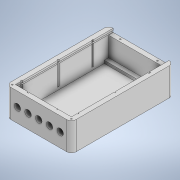
# Autodesk Inventor part: carcasa inferior
Saved by Autodesk Inventor 2020 (Build 240168000, 168)
## iProperties
Created: 2022-05-20
Part Number: carcasa inferior
Material: Generic
Document SubType Name: Modeling
Designer: juanc
Density: 1 g/cm^3
Appearance: Default
Author: juanc
## iProperties of the stored document _3DPrint.ipt
Created: 2022-05-23
Part Number: _3DPrint
Material: Generic
Document SubType Name: Modeling
Designer: juanc
Density: 1 g/cm^3
Appearance: Default
Author: juanc
Autodesk Inventor part; units mm, degrees
ref_plane "YZ Plane" through (0, 0, 0) normal (1, 0, 0) x (0, 1, 0)
ref_plane "XZ Plane" through (0, 0, 0) normal (0, 1, 0) x (-1, 0, 0)
sketch "Sketch1" plane through (0, 0, 0) normal (0, 1, 0) x (-1, 0, 0)
  line L0 (0, 0) -> (60, 0)
  line L1 (60, 0) -> (60, -100)
  line L2 (60, -100) -> (0, -100)
  line L3 (0, -100) -> (0, 0)
  line L4 (60, 0) -> (0, -100) construction
  line L5 (60, -100) -> (0, 0) construction
  line L6 (-5, 5) -> (65, 5)
  line L7 (65, 5) -> (65, -105)
  line L8 (65, -105) -> (-5, -105)
  line L9 (-5, -105) -> (-5, 5)
  line L10 (-5, 5) -> (65, -105) construction
  line L11 (65, 5) -> (-5, -105) construction
  point P0 (30, -50)
  dimension "d0" = 60
  dimension "d1" = 100
  dimension "d2" = 70
  dimension "d3" = 110
  constraints: 24 end point, 4 parallel, 3 midpoint, 2 horizontal, 2 perpendicular
  measures "d0" distance of L1.end L2.end
  measures "d1" distance of L0.end L1.end
  measures "d2" distance of L7.end L8.end
  measures "d3" distance of L6.end L7.end
extrude "Extrusion1" add sketch "Sketch1" along normal blind 30
extrude "Extrusion2" add sketch "Sketch1" along normal blind 5 contours L0 L1 L2 L3
fillet "Fillet1" radius 5 4 edges at (5, 15, 5) (-65, 15, 5) (5, 15, -105) (-65, 15, -105)
sketch "Sketch2" plane through (0, 0, -105) normal (0, 0, -1) x (-1, 0, 0)
  line L0 (60, 30) -> (0, 30) construction
  line L1 (60, 5) -> (60, 30) construction
  line L2 (0, 30) -> (60, 30) construction
  line L3 (60, 30) -> (60, 26) construction
  line L4 (60, 26) -> (0, 26) construction
  line L5 (0, 26) -> (0, 30) construction
  line L6 (0, 30) -> (60, 30)
  line L7 (60, 30) -> (60, 26)
  line L8 (60, 26) -> (0, 26)
  line L9 (0, 26) -> (0, 30)
  point P0 (0, 0)
  dimension "d9" = 4
  constraints: 16 end point, 4 parallel, 2 horizontal, 2 perpendicular, 1 point on line
  measures "d9" distance of L2.end L3.end
extrude "Extrusion3" cut sketch "Sketch2" against normal blind 10
ref_plane "Work Plane1" through (0, 0, -105.25) normal (0, 0, -1) x (-1, 0, 0)
sketch "Sketch3" plane through (0, 0, -105.25) normal (0, 0, -1) x (-1, 0, 0)
  line L0 (-5, 30) -> (0, 30) construction
  line L1 (0, 30) -> (0, 28) construction
  line L2 (0, 26) -> (60, 26) construction
  line L3 (0, 28) -> (60, 28) construction
  line L4 (0, 28) -> (0, 26.5) construction
  line L5 (0, 5) -> (0, 30) construction
  line L6 (0, 28) -> (-1.5, 28) construction
  line L7 (-1.5, 28) -> (61.5, 28)
  line L8 (61.5, 28) -> (61.5, 26.5)
  line L9 (61.5, 26.5) -> (-1.5, 26.5)
  line L10 (-1.5, 26.5) -> (-1.5, 28)
  point P0 (0, 0)
  dimension "d17" = 2
  dimension "d19" = 1.5
  dimension "d20" = 63
  dimension "d21" = 1.5
  constraints: 16 end point, 3 parallel, 2 horizontal, 2 perpendicular, 1 point on line
  measures "d17" distance of L0.end L1.end
  measures "d19" distance of L1.end L6.end
  measures "d20" distance of L8.end L9.end
  measures "d21" distance of L7.end L8.end
extrude "Extrusion4" cut sketch "Sketch3" against normal blind 105
sketch "Sketch4" plane through (0, 5, 0) normal (0, 1, 0) x (1, 0, 0)
  line L0 (-60, 0) -> (-60, 100) projected
  line L1 (-60, 95.3368) -> (-19, 95.3368)
  line L2 (-19, 95.3368) -> (-19, 22.3368)
  line L3 (-19, 22.3368) -> (-60, 22.3368)
  line L4 (-60, 22.3368) -> (-60, 95.3368)
  point P0 (0, 0)
  dimension "d24" = 41
  dimension "d25" = 73
  constraints: 8 end point, 2 parallel, 1 horizontal, 1 perpendicular, 1 point on line
  measures "d24" distance of L2.end L3.end
  measures "d25" distance of L1.end L2.end
extrude "Extrusion5" cut sketch "Sketch4" against normal blind 3
sketch "Sketch5" plane through (-60, 0, 5) normal (0, 0, 1) x (1, 0, 0)
  line L0 (60, 30) -> (0, 30) construction
  line L1 (65, 0) -> (60, 0) construction
  line L2 (60, 0) -> (60, 30) construction
  line L3 (0, 0) -> (-5, 0) construction
  line L4 (0, 5) -> (0, 30) projected
  line L5 (60, 30) -> (60, 0) projected
  line L6 (0, 15) -> (7, 15) construction
  line L7 (60, 15) -> (53, 15) construction
  line L8 (7, 15) -> (53, 15) construction
  line L9 (18.5, 15) -> (64.5, 15) construction
  line L10 (30, 15) -> (76, 15) construction
  line L11 (41.5, 15) -> (87.5, 15) construction
  line L12 (53, 15) -> (99, 15) construction
  dimension "d28" = 7
  dimension "d29" = 7
  dimension "d32" = 11.5
  constraints: 16 end point, 5 coincident, 2 collinear, 1 horizontal, 1 midpoint, 1 perpendicular, 1 point on line, 15 other
  measures "d28" distance of L6.start L6.end
  measures "d29" distance of L7.start L7.end
  measures "d32" distance of point (7, 15) point (18.5, 15)
hole "Hole1" at (-53, 15, 5) at (-41.5, 15, 5) at (-30, 15, 5) at (-18.5, 15, 5) at (-7, 15, 5) direction (0, 0, -1) diameter 7 depth 8 tip angle 118
sketch "Sketch7" plane through (0, 0, 0) normal (0, -1, 0) x (1, 0, 0)
  line L0 (0, 0) -> (-60, 0) construction
  line L1 (0, 0) -> (1.7678, 1.7678) construction
  line L2 (0, 0) -> (2.5, 0) construction
  line L3 (-60, 0) -> (-61.7678, 1.7678) construction
  line L4 (-60, 0) -> (-57.5, 0) construction
  dimension "d55" = 2.5
  dimension "d56" = 45
  dimension "d57" = 2.5
  dimension "d58" = 135
  constraints: 8 end point, 2 coincident, 2 equal length, 2 horizontal
  measures "d55" distance of L0.start L1.end
  measures "d56" angle of L2 L1
  measures "d57" distance of L0.end L3.end
  measures "d58" angle of L4 L3
hole "Hole3" at (1.7678, 0, 1.7678) at (-61.7678, 0, 1.7678) direction (0, 1, 0) diameter 1.5 depth 40 tip angle 118 counterbore diameter 2.5 counterbore depth 1
sketch "Sketch8" plane through (0, 0, 0) normal (0, -1, 0) x (1, 0, 0)
  line L0 (0, -105) -> (0, 0) construction
  arc A0 (-61.5, -104.7697) -> (-60, -105) centre (-60, -100) ccw construction
  line L1 (-60, -105) -> (0, -105) construction
  line L2 (-30, -102.5) -> (0, -102.5) construction
  line L3 (-30, -102.5) -> (-60, -102.5) construction
  line L4 (-60, -105) -> (-60, -100) construction
  line L5 (-30, -102.5) -> (-50, -102.5) construction
  line L6 (-30, -102.5) -> (-10, -102.5) construction
  line L7 (-30, -102.5) -> (-10, -102.5) construction
  dimension "d66" = 20
  dimension "d67" = 180
  dimension "d68" = 20
  constraints: 10 end point, 3 collinear, 2 coincident, 1 horizontal, 1 midpoint, 1 perpendicular, 1 point on line
  measures "d66" distance of L2.start L5.end
  measures "d67" angle of L5 L6
  measures "d68" distance of L2.start L6.end
hole "Hole4" at (-50, 0, -102.5) at (-10, 0, -102.5) direction (0, 1, 0) diameter 1.5 depth 40 tip angle 118 counterbore diameter 2.5 counterbore depth 1
sketch "Sketch9" plane through (0, 30, 0) normal (0, 1, 0) x (1, 0, 0)
  line L0 (0, 105) -> (0, 0) construction
  line L1 (0, 0) -> (1, 0) construction
  line L2 (1, 0) -> (1, 100) construction
  line L3 (1, 5.7254) -> (-61, 5.7254)
  line L4 (-61, 5.7254) -> (-61, 7.7254)
  line L5 (-61, 7.7254) -> (1, 7.7254)
  line L6 (1, 7.7254) -> (1, 5.7254)
  dimension "d76" = 1
  dimension "d77" = 100
  dimension "d78" = 62
  dimension "d79" = 2
  constraints: 12 end point, 3 parallel, 2 horizontal, 1 perpendicular, 1 point on line
  measures "d76" distance of L0.end L1.end
  measures "d77" distance of L1.end L2.end
  measures "d78" distance of L4.end L5.end
  measures "d79" distance of L3.end L4.end
extrude "Extrusion6" cut sketch "Sketch9" against normal blind 25
fillet "Fillet2" radius 1 4 edges at (1, 29, -5.7254) (1, 29, -7.7254) (1, 15.75, -5.7254) (1, 15.75, -7.7254)
fillet "Fillet3" radius 1 4 edges at (-61, 15.75, -5.7254) (-61, 29, -5.7254) (-61, 29, -7.7254) (-61, 15.75, -7.7254)
sketch "Sketch10" plane through (0, 30, 0) normal (0, 1, 0) x (1, 0, 0)
  arc A0 (0, 5.7254) -> (0, 7.7254) centre (0, 6.7254) ccw construction
  line L0 (1, 6.7254) -> (1, 94.9249) construction
  line L1 (1, 47) -> (-61, 47)
  line L2 (-61, 47) -> (-61, 45)
  line L3 (-61, 45) -> (1, 45)
  line L4 (1, 45) -> (1, 47)
  line L5 (1.5, 104.7697) -> (1.5, 0.25) projected
  line L6 (1.5, 84) -> (-60.5, 84)
  line L7 (-60.5, 84) -> (-60.5, 82)
  line L8 (-60.5, 82) -> (1.5, 82)
  line L9 (1.5, 82) -> (1.5, 84)
  line L10 (-1.7037, 82) -> (-1.7037, 47) construction
  line L11 (-14.6781, 45) -> (-14.6781, 0) construction
  line L12 (0, 0) -> (-60, 0) construction
  line L13 (0, 6.7254) -> (20.1927, 45) construction
  point P0 (1.5, 82)
  dimension "d84" = 62
  dimension "d85" = 2
  dimension "d86" = 62
  dimension "d87" = 2
  dimension "d88" = 35
  dimension "d90" = 45
  dimension "d91" = 43.2746
  constraints: 24 end point, 7 point on line, 4 parallel, 3 perpendicular, 2 horizontal, 1 point on circle, 1 vertical
  measures "d84" distance of L3.end L2.end
  measures "d85" distance of L2.end L1.end
  measures "d86" distance of L8.end L7.end
  measures "d87" distance of L7.end L6.end
  measures "d88" distance of L10.start L10.end
  measures "d90" distance of L11.start L11.end
  measures "d91" distance of L13.start L13.end
extrude "Extrusion7" cut sketch "Sketch10" against normal blind 25
fillet "Fillet4" radius 1 8 edges at (1, 29, -45) (1, 29, -47) (1, 15.75, -47) (1, 15.75, -45) (1.5, 29, -82) (1.5, 29, -84) (1.5, 15.75, -82) (1.5, 15.75, -84)
fillet "Fillet5" radius 1 8 edges at (-61, 15.75, -47) (-61, 15.75, -45) (-61, 29, -47) (-61, 29, -45) (-60.5, 15.75, -84) (-60.5, 15.75, -82) (-60.5, 29, -84) (-60.5, 29, -82)
sketch "Sketch11" plane through (0, 30, 0) normal (0, 1, 0) x (1, 0, 0)
  line L0 (-60, 0.25) -> (-60, 5.7254) projected
  line L1 (-60, 0.25) -> (-60, -0.75)
  line L2 (-13, -0.75) -> (-15, -0.75)
  line L3 (-15, -0.75) -> (-15, 1.25)
  line L4 (-15, 1.25) -> (-13, 1.25)
  line L5 (-13, 1.25) -> (-13, -0.75)
  line L6 (-13, 1.25) -> (0, 1.25) construction
  line L7 (0, 5.7254) -> (0, 0) construction
  line L8 (-60, 0) -> (-60, 5.7254) construction
  line L9 (-60, 0) -> (-47, 0) construction
  line L10 (0, 0) -> (-60, 0) construction
  line L11 (-47, 0) -> (-45, 0)
  line L12 (-45, 0) -> (-45, -1)
  line L13 (-45, -1) -> (-47, -1)
  line L14 (-47, -1) -> (-47, 0)
  dimension "d96" = 1
  dimension "d97" = 2
  dimension "d98" = 2
  dimension "d100" = 13
  dimension "d101" = 13
  dimension "d102" = 2
  dimension "d103" = 1
  constraints: 22 end point, 4 parallel, 3 horizontal, 2 perpendicular, 2 point on line, 1 collinear
  measures "d96" distance of L0.start L1.end
  measures "d97" distance of L3.end L4.end
  measures "d98" distance of L2.end L3.end
  measures "d100" distance of L4.end L6.end
  measures "d101" distance of L8.start L9.end
  measures "d102" distance of L12.end L13.end
  measures "d103" distance of L11.end L12.end
extrude "Extrusion8" cut sketch "Sketch11" against normal blind 25
fillet "Fillet6" radius 1 2 edges at (-47, 17.5, 1) (-13, 17.5, 0.75)
body "Solid1"
